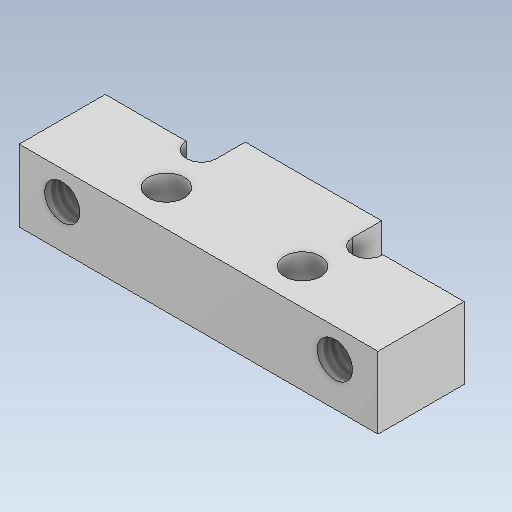
# Autodesk Inventor part: Foot_root_block
Saved by Autodesk Inventor 2020.4 (Build 244396000, 396)
## iProperties
Created: 2021-09-15
Part Number: Foot_root_block
Material: アルミニウム 2014-T4
Document SubType Name: Modeling
Designer: naoki
Density: 2.8 g/cm^3
Appearance: 滑らか - 淡い灰色
Description: A2017 T5
Author: naoki
Autodesk Inventor part; units mm, degrees
ref_plane "YZ Plane" through (0, 0, 0) normal (1, 0, 0) x (0, 1, 0)
ref_plane "XZ Plane" through (0, 0, 0) normal (0, 1, 0) x (-1, 0, 0)
ref_plane "XY Plane" through (0, 0, 0) normal (0, 0, 1) x (1, 0, 0)
derived "Foot_back_frame.ipt"
sketch "スケッチ1" plane through (0, 0, 0) normal (0, 0, 1) x (1, 0, 0)
  line L0 (-63.6765, 0) -> (66.53, 0) construction
  line L1 (0, 73.5962) -> (0, -63.7716) construction
  circle A0 centre (0, 0) radius 5.05 construction
  circle A1 centre (0, 0) radius 8 construction
  circle A2 centre (0, 0) radius 11.25 construction
  circle A3 centre (0, 8.5) radius 1.35 construction
  circle A4 centre (0, 8.5) radius 2.75 construction
  circle A5 centre (-8.5, 0) radius 2.75 construction
  circle A6 centre (-8.5, 0) radius 1.35 construction
  circle A7 centre (0, -8.5) radius 2.75 construction
  circle A8 centre (0, -8.5) radius 1.35 construction
  circle A9 centre (8.5, 0) radius 2.75 construction
  circle A10 centre (8.5, 0) radius 1.35 construction
  line L2 (12.5, -41) -> (-12.5, -41)
  line L3 (-12.5, -41) -> (-12.5, -36)
  line L4 (-12.5, -36) -> (12.5, -36)
  line L5 (12.5, -36) -> (12.5, -41)
  line L6 (12.5, -41) -> (-12.5, -36) construction
  line L7 (-12.5, -41) -> (12.5, -36) construction
  line L8 (12.5, -36) -> (11.2433, 0.3883) construction
  line L9 (-12.5, -36) -> (-11.2433, 0.3883) construction
  circle A11 centre (-9.5, -38) radius 1.55
  line L10 (-12.5, -38) -> (12.5, -38)
  line L11 (-4.75, -36) -> (-4.75, -41) construction
  line L12 (4.75, -36) -> (4.75, -41) construction
  circle A12 centre (9.5, -38) radius 1.55
  line L13 (-4.75, -36) -> (4.75, -36) construction
  line L14 (4.75, -36) -> (4.75, -38.5)
  line L15 (4.75, -38.5) -> (-4.75, -38.5)
  line L16 (-4.75, -38.5) -> (-4.75, -36)
  line L17 (-4.75, -37.25) -> (4.75, -37.25) construction
  line L18 (-4.76, -38.51) -> (4.76, -38.51) construction
  line L19 (4.76, -38.51) -> (4.76, -35.99) construction
  line L20 (4.76, -35.99) -> (-4.76, -35.99) construction
  line L21 (-4.76, -35.99) -> (-4.76, -38.51) construction
  circle A13 centre (-3.71, -35.99) radius 1.05
  circle A14 centre (-3.71, -38.51) radius 1.05
  circle A15 centre (3.71, -38.51) radius 1.05
  circle A16 centre (3.71, -35.99) radius 1.05
  point P0 (0, -38.5)
  point P1 (4.75, -36)
  point P2 (4.75, -38)
  point P3 (-4.75, -38)
  point P4 (2.66, -38.51)
  point P5 (-2.66, -38.51)
  point P6 (-2.66, -35.99)
  point P7 (2.66, -35.99)
  dimension "d12" = 7.75
  dimension "d13" = 7.75
  measures "d12" distance between parallel lines of L5 L12
  measures "d13" distance between parallel lines of L3 L16
extrude "押し出し1" add sketch "スケッチ1" along normal blind 6 contours L2 L3 L10 A11 L16 A14 L15 A15 L14 A12 L5 | L10 A12 L14 A16 L4 L5 | L3 L4 A13 L16 L10 A11 | A12 L10 | L10 A12 | L10 A11 | A11 L10 | A16 L14 L4 | L4 L16 A13 | L14 A16 L4 | L14 L10 A15 A14 L16 A13 L4 A16 | L14 A15 L10 | L4 A13 L16 | L10 A14 L16 | A15 L14 L15 L10 | L10 A15 | A15 L15 L14 | A14 L10 | L10 A14 L15 L16 | L16 L15 A14 | A15 L15 A14 L10
extrude "押し出し2" add sketch "スケッチ1" against normal blind 2 contours L14 A16 L4 | L14 L10 A15 A14 L16 A13 L4 A16 | L14 A15 L10 | L4 A13 L16 | L10 A14 L16 | A15 L14 L15 L10 | L10 A15 | A14 L10 | L10 A14 L15 L16 | A15 L15 A14 L10 picked at (3.3684, -36.0863) picked at (-3.3684, -36.0863)
hole "穴1" at (9.5, -38, 0) at (-9.5, -38, 0) direction (0, 0, 1) diameter 2.459 end through all thread size "M3x0.5" class "6H" standard "ANSI Metric M Profile"
sketch "スケッチ3" plane through (-12.5, -41, 0) normal (0, -1, 0) x (1, 0, 0)
  line L0 (0, 0) -> (25, 0) projected
  line L1 (17.25, 0) -> (17.25, -2) projected
  arc A0 (19.35, 0) -> (17.25, 0) centre (18.3, 0) ccw
  line L2 (7.75, 0) -> (0, 0) projected
  arc A1 (7.75, 0) -> (5.65, 0) centre (6.7, 0) ccw
  line L3 (25, 0) -> (25, 6) projected
  line L4 (0, 0) -> (0, 6) projected
  point P0 (12.5, 0)
  point P1 (19.35, 0)
  point P2 (17.25, 3.5)
  point P3 (7.75, 3.5)
  dimension "d20" = 1.05
  dimension "d23" = 1.05
  dimension "d24" = 7.75
  dimension "d25" = 7.75
  dimension "d26" = 3.5
  dimension "d27" = 3.5
  constraints: 4 point on circle, 2 centre point, 2 point on line
  measures "d20" radius of A0
  measures "d23" radius of A1
  measures "d24" distance from line of L3 point (17.25, 3.5)
  measures "d25" distance from line of L4 point (7.75, 3.5)
  measures "d26" distance from line of L0 point (17.25, 3.5)
  measures "d27" distance from line of L0 point (7.75, 3.5)
extrude "押し出し3" cut sketch "スケッチ3" against normal blind 5
hole "穴2" at (4.75, -41, 3.5) at (-4.75, -41, 3.5) direction (0, 1, 0) diameter 2.5 end through all
equation "\"d23\" = d20"
equation "\"d25\" = d24"
equation "\"d27\" = d26"
